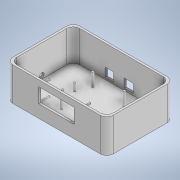
# Autodesk Inventor part: krabička
Saved by Autodesk Inventor 2021 (Build 250183000, 183)
## iProperties
Created: 2020-12-02
Part Number: krabička
Material: Všeobecné
Document SubType Name: Modeling
Designer: Adam
Density: 1 g/cm^3
Appearance: Výchozí
Author: Adam
Autodesk Inventor part; units mm, degrees
ref_plane "YZ Plane" through (0, 0, 0) normal (1, 0, 0) x (0, 1, 0)
ref_plane "XZ Plane" through (0, 0, 0) normal (0, 1, 0) x (-1, 0, 0)
ref_plane "XY Plane" through (0, 0, 0) normal (0, 0, 1) x (1, 0, 0)
sketch "Náčrt1" plane through (0, 0, 0) normal (0, 1, 0) x (-1, 0, 0)
  line L0 (0, 0) -> (-150, 0)
  line L1 (-150, 0) -> (-150, -100)
  line L2 (-150, -100) -> (0, -100)
  line L3 (0, -100) -> (0, 0)
  dimension "d0" = 150
  dimension "d1" = 100
  constraints: 8 end point, 2 parallel, 1 horizontal, 1 perpendicular
  measures "d0" distance of L1.end L2.end
  measures "d1" distance of L0.end L1.end
extrude "Vysunutí1" add sketch "Náčrt1" along normal blind 50
sketch "Náčrt2" plane through (0, 50, 0) normal (0, 1, 0) x (1, 0, 0)
  line L0 (3, 97) -> (147, 97)
  line L1 (147, 97) -> (147, 3)
  line L2 (147, 3) -> (3, 3)
  line L3 (3, 3) -> (3, 97)
  line L4 (0, 100) -> (0, 0) projected
  line L5 (150, 100) -> (0, 100) projected
  dimension "d4" = 144
  dimension "d5" = 94
  dimension "d6" = 3
  dimension "d7" = 3
  constraints: 8 end point, 2 parallel, 1 horizontal, 1 perpendicular
  measures "d4" distance of L0.start L0.end
  measures "d5" distance of L0.end L1.end
  measures "d6" distance between parallel lines of L4 L3
  measures "d7" distance between parallel lines of L5 L0
extrude "Vysunutí2" cut sketch "Náčrt2" against normal blind 47
sketch "Náčrt3" plane through (0, 0, 0) normal (0, 0, 1) x (1, 0, 0)
  line L0 (48.5, 41) -> (101.5, 41)
  line L1 (101.5, 41) -> (101.5, 19)
  line L2 (101.5, 19) -> (48.5, 19)
  line L3 (48.5, 19) -> (48.5, 41)
  line L4 (0, 0) -> (0, 50) projected
  line L5 (0, 0) -> (150, 0) projected
  dimension "d10" = 22
  dimension "d11" = 53
  dimension "d12" = 48.5
  dimension "d13" = 19
  constraints: 8 end point, 2 parallel, 1 horizontal, 1 perpendicular
  measures "d10" distance of L0.end L1.end
  measures "d11" distance of L1.end L2.end
  measures "d12" distance between parallel lines of L4 L3
  measures "d13" distance between parallel lines of L5 L2
extrude "Vysunutí3" cut sketch "Náčrt3" against normal blind 3
sketch "Náčrt4" plane through (147, 50, -3) normal (0, 0, -1) x (-1, 0, 0)
  line L0 (37.5, -7.5) -> (103.5, -7.5)
  line L1 (103.5, -7.5) -> (103.5, -34.5)
  line L2 (103.5, -34.5) -> (37.5, -34.5)
  line L3 (37.5, -34.5) -> (37.5, -7.5)
  line L4 (98.5, -9) -> (98.5, -31) projected
  line L5 (98.5, -31) -> (45.5, -31) projected
  circle A0 centre (101, -10) radius 1.5
  circle A1 centre (40, -10) radius 1.5
  circle A2 centre (40, -32) radius 1.5
  circle A3 centre (101, -32) radius 1.5
  line L6 (45.5, -31) -> (45.5, -9) projected
  line L7 (46.5, -10.5) -> (97.5, -10.5)
  line L8 (97.5, -10.5) -> (97.5, -29.5)
  line L9 (97.5, -29.5) -> (46.5, -29.5)
  line L10 (46.5, -29.5) -> (46.5, -10.5)
  line L11 (45.5, -9) -> (98.5, -9) projected
  point P0 (147, -50)
  point P1 (98.5, -37)
  dimension "d16" = 66
  dimension "d17" = 27
  dimension "d19" = 3.5
  dimension "d21" = 3
  dimension "d22" = 3
  dimension "d23" = 3
  dimension "d24" = 3
  dimension "d56" = 1
  dimension "d57" = 1
  dimension "d58" = 1
  dimension "d59" = 1
  dimension "d60" = 1
  dimension "d61" = 1
  dimension "d62" = 1
  dimension "d63" = 1
  dimension "d129" = 1
  dimension "d130" = 51
  dimension "d131" = 19
  dimension "d132" = 1.5
  dimension "d133" = 6
  dimension "d134" = 9
  constraints: 16 end point, 4 centre point, 3 parallel, 2 horizontal, 2 perpendicular
  measures "d16" distance of L0.start L0.end
  measures "d17" distance of L0.end L1.end
  measures "d19" distance between parallel lines of L5 L2
  measures "d21" diameter of A0
  measures "d22" diameter of A1
  measures "d23" diameter of A2
  measures "d24" diameter of A3
  measures "d56" distance edge to line of A0 L0
  measures "d57" distance edge to line of A0 L1
  measures "d58" distance edge to line of A3 L1
  measures "d59" distance edge to line of A3 L2
  measures "d60" distance edge to line of A1 L0
  measures "d61" distance edge to line of A1 L3
  measures "d62" distance edge to line of A2 L3
  measures "d63" distance edge to line of A2 L2
  measures "d129" distance between parallel lines of L6 L10
  measures "d130" distance of L7.start L7.end
  measures "d131" distance of L7.end L8.end
  measures "d132" distance between parallel lines of L7 L11
  measures "d133" distance between parallel lines of L8 L1
  measures "d134" distance between parallel lines of L3 L10
extrude "Vysunutí4" add sketch "Náčrt4" along normal blind 15 contours A0 | A1 | A2 | A3
fillet "Zaoblení1" radius 10 8 edges at (150, 25, 0) (150, 25, -100) (3, 26.5, -97) (0, 25, -100) (0, 25, 0) (3, 26.5, -3) (147, 26.5, -3) (147, 26.5, -97)
sketch "Náčrt7" plane through (0, 3, 0) normal (0, 1, 0) x (1, 0, 0)
  line L0 (137, 3) -> (13, 3) projected
  line L1 (150, 10) -> (150, 90) projected
  line L2 (13, 97) -> (137, 97) projected
  line L3 (101.7363, 91.2274) -> (101.7363, 27.7499)
  line L4 (101.694, 91.4813) -> (101.7363, 91.2274)
  line L5 (101.5882, 91.7141) -> (101.694, 91.4813)
  line L6 (101.44, 91.9257) -> (101.5882, 91.7141)
  line L7 (101.2285, 92.095) -> (101.44, 91.9257)
  line L8 (100.9957, 92.1796) -> (101.2285, 92.095)
  line L9 (100.7206, 92.2219) -> (100.9957, 92.1796)
  line L10 (49.4308, 92.2219) -> (100.7206, 92.2219)
  line L11 (49.1768, 92.1796) -> (49.4308, 92.2219)
  line L12 (48.9441, 92.095) -> (49.1768, 92.1796)
  line L13 (48.7325, 91.9257) -> (48.9441, 92.095)
  line L14 (48.5632, 91.7141) -> (48.7325, 91.9257)
  line L15 (48.4786, 91.4813) -> (48.5632, 91.7141)
  line L16 (48.4363, 91.2274) -> (48.4786, 91.4813)
  line L17 (48.4363, 27.2968) -> (48.4363, 91.3033)
  line L18 (48.4786, 26.967) -> (48.4363, 27.2209)
  line L19 (48.5632, 26.7342) -> (48.4786, 26.967)
  line L20 (48.7325, 26.5226) -> (48.5632, 26.7342)
  line L21 (48.9441, 26.3533) -> (48.7325, 26.5226)
  line L22 (49.1768, 26.2687) -> (48.9441, 26.3533)
  line L23 (49.4308, 26.2264) -> (49.1768, 26.2687)
  line L24 (50.9754, 26.2264) -> (49.4308, 26.2264)
  line L25 (53.5145, 23.6873) -> (50.9754, 26.2264)
  line L26 (86.2836, 23.6873) -> (53.5504, 23.6873)
  line L27 (88.7869, 26.2264) -> (86.2477, 23.6873)
  line L28 (100.2128, 26.2264) -> (88.7869, 26.2264)
  line L29 (101.7363, 27.7499) -> (100.2128, 26.2264)
  line L30 (97.5901, 76.9312) -> (97.593, 76.8751)
  line L31 (97.593, 76.8751) -> (97.5979, 76.8192)
  line L32 (97.5979, 76.8192) -> (97.6047, 76.7635)
  line L33 (97.6047, 76.7635) -> (97.6135, 76.708)
  line L34 (97.6135, 76.708) -> (97.6242, 76.6529)
  line L35 (97.6242, 76.6529) -> (97.6368, 76.5983)
  line L36 (97.6368, 76.5983) -> (97.6514, 76.544)
  line L37 (97.6514, 76.544) -> (97.6678, 76.4904)
  line L38 (97.6678, 76.4904) -> (97.6861, 76.4373)
  line L39 (97.6861, 76.4373) -> (97.7062, 76.3849)
  line L40 (97.7062, 76.3849) -> (97.7281, 76.3332)
  line L41 (97.7281, 76.3332) -> (97.7518, 76.2823)
  line L42 (97.7518, 76.2823) -> (97.7773, 76.2323)
  line L43 (97.7773, 76.2323) -> (97.8045, 76.1832)
  line L44 (97.8045, 76.1832) -> (97.8334, 76.1351)
  line L45 (97.8334, 76.1351) -> (97.864, 76.0881)
  line L46 (97.864, 76.0881) -> (97.8962, 76.0421)
  line L47 (97.8962, 76.0421) -> (97.93, 75.9972)
  line L48 (97.93, 75.9972) -> (97.9653, 75.9536)
  line L49 (97.9653, 75.9536) -> (98.0021, 75.9113)
  line L50 (98.0021, 75.9113) -> (98.0404, 75.8702)
  line L51 (98.0404, 75.8702) -> (98.0801, 75.8305)
  line L52 (98.0801, 75.8305) -> (98.1211, 75.7922)
  line L53 (98.1211, 75.7922) -> (98.1635, 75.7554)
  line L54 (98.1635, 75.7554) -> (98.2071, 75.7201)
  line L55 (98.2071, 75.7201) -> (98.252, 75.6863)
  line L56 (98.252, 75.6863) -> (98.2979, 75.6541)
  line L57 (98.2979, 75.6541) -> (98.345, 75.6235)
  line L58 (98.345, 75.6235) -> (98.3931, 75.5946)
  line L59 (98.3931, 75.5946) -> (98.4422, 75.5674)
  line L60 (98.4422, 75.5674) -> (98.4922, 75.5419)
  line L61 (98.4922, 75.5419) -> (98.5431, 75.5182)
  line L62 (98.5431, 75.5182) -> (98.5948, 75.4963)
  line L63 (98.5948, 75.4963) -> (98.6472, 75.4762)
  line L64 (98.6472, 75.4762) -> (98.7002, 75.4579)
  line L65 (98.7002, 75.4579) -> (98.7539, 75.4415)
  line L66 (98.7539, 75.4415) -> (98.8081, 75.427)
  line L67 (98.8081, 75.427) -> (98.8628, 75.4143)
  line L68 (98.8628, 75.4143) -> (98.9179, 75.4036)
  line L69 (98.9179, 75.4036) -> (98.9734, 75.3948)
  line L70 (98.9734, 75.3948) -> (99.0291, 75.388)
  line L71 (99.0291, 75.388) -> (99.085, 75.3831)
  line L72 (99.085, 75.3831) -> (99.1411, 75.3802)
  line L73 (99.1411, 75.3802) -> (99.1972, 75.3792)
  line L74 (99.1972, 75.3792) -> (99.2529, 75.3802)
  line L75 (99.2529, 75.3802) -> (99.3085, 75.3831)
  line L76 (99.3085, 75.3831) -> (99.364, 75.3879)
  line L77 (99.364, 75.3879) -> (99.4193, 75.3946)
  line L78 (99.4193, 75.3946) -> (99.4744, 75.4033)
  line L79 (99.4744, 75.4033) -> (99.5291, 75.4138)
  line L80 (99.5291, 75.4138) -> (99.5834, 75.4263)
  line L81 (99.5834, 75.4263) -> (99.6373, 75.4406)
  line L82 (99.6373, 75.4406) -> (99.6906, 75.4568)
  line L83 (99.6906, 75.4568) -> (99.7433, 75.4748)
  line L84 (99.7433, 75.4748) -> (99.7954, 75.4946)
  line L85 (99.7954, 75.4946) -> (99.8467, 75.5162)
  line L86 (99.8467, 75.5162) -> (99.8973, 75.5396)
  line L87 (99.8973, 75.5396) -> (99.947, 75.5647)
  line L88 (99.947, 75.5647) -> (99.9959, 75.5916)
  line L89 (99.9959, 75.5916) -> (100.0437, 75.6201)
  line L90 (100.0437, 75.6201) -> (100.0906, 75.6502)
  line L91 (100.0906, 75.6502) -> (100.1364, 75.682)
  line L92 (100.1364, 75.682) -> (100.181, 75.7153)
  line L93 (100.181, 75.7153) -> (100.2245, 75.7501)
  line L94 (100.2245, 75.7501) -> (100.2667, 75.7865)
  line L95 (100.2667, 75.7865) -> (100.3077, 75.8242)
  line L96 (100.3077, 75.8242) -> (100.3473, 75.8634)
  line L97 (100.3473, 75.8634) -> (100.3856, 75.9039)
  line L98 (100.3856, 75.9039) -> (100.4224, 75.9457)
  line L99 (100.4224, 75.9457) -> (100.4577, 75.9888)
  line L100 (100.4577, 75.9888) -> (100.4916, 76.0331)
  line L101 (100.4916, 76.0331) -> (100.5239, 76.0785)
  line L102 (100.5239, 76.0785) -> (100.5545, 76.125)
  line L103 (100.5545, 76.125) -> (100.5836, 76.1725)
  line L104 (100.5836, 76.1725) -> (100.611, 76.2211)
  line L105 (100.611, 76.2211) -> (100.6367, 76.2705)
  line L106 (100.6367, 76.2705) -> (100.6607, 76.3208)
  line L107 (100.6607, 76.3208) -> (100.6829, 76.3719)
  line L108 (100.6829, 76.3719) -> (100.7033, 76.4237)
  line L109 (100.7033, 76.4237) -> (100.7219, 76.4763)
  line L110 (100.7219, 76.4763) -> (100.7387, 76.5294)
  line L111 (100.7387, 76.5294) -> (100.7536, 76.5831)
  line L112 (100.7536, 76.5831) -> (100.7667, 76.6372)
  line L113 (100.7667, 76.6372) -> (100.7779, 76.6918)
  line L114 (100.7779, 76.6918) -> (100.7872, 76.7467)
  line L115 (100.7872, 76.7467) -> (100.7946, 76.802)
  line L116 (100.7946, 76.802) -> (100.8, 76.8574)
  line L117 (100.8, 76.8574) -> (100.8036, 76.913)
  line L118 (100.8036, 76.913) -> (100.8052, 76.9687)
  line L119 (100.8052, 76.9687) -> (100.8048, 77.0244)
  line L120 (100.8048, 77.0244) -> (100.8026, 77.0801)
  line L121 (100.8026, 77.0801) -> (100.7984, 77.1357)
  line L122 (100.7984, 77.1357) -> (100.7923, 77.1911)
  line L123 (100.7923, 77.1911) -> (100.7843, 77.2462)
  line L124 (100.7843, 77.2462) -> (100.7744, 77.301)
  line L125 (100.7744, 77.301) -> (100.7626, 77.3555)
  line L126 (100.7626, 77.3555) -> (100.7489, 77.4095)
  line L127 (100.7489, 77.4095) -> (100.7333, 77.463)
  line L128 (100.7333, 77.463) -> (100.7159, 77.5159)
  line L129 (100.7159, 77.5159) -> (100.6967, 77.5682)
  line L130 (100.6967, 77.5682) -> (100.6757, 77.6198)
  line L131 (100.6757, 77.6198) -> (100.6529, 77.6706)
  line L132 (100.6529, 77.6706) -> (100.6283, 77.7207)
  line L133 (100.6283, 77.7207) -> (100.602, 77.7698)
  line L134 (100.602, 77.7698) -> (100.5741, 77.818)
  line L135 (100.5741, 77.818) -> (100.5445, 77.8652)
  line L136 (100.5445, 77.8652) -> (100.5133, 77.9113)
  line L137 (100.5133, 77.9113) -> (100.4805, 77.9564)
  line L138 (100.4805, 77.9564) -> (100.4461, 78.0003)
  line L139 (100.4461, 78.0003) -> (100.4103, 78.0429)
  line L140 (100.4103, 78.0429) -> (100.373, 78.0843)
  line L141 (100.373, 78.0843) -> (100.3343, 78.1244)
  line L142 (100.3343, 78.1244) -> (100.2942, 78.1631)
  line L143 (100.2942, 78.1631) -> (100.2528, 78.2004)
  line L144 (100.2528, 78.2004) -> (100.2101, 78.2362)
  line L145 (100.2101, 78.2362) -> (100.1663, 78.2706)
  line L146 (100.1663, 78.2706) -> (100.1212, 78.3034)
  line L147 (100.1212, 78.3034) -> (100.0751, 78.3346)
  line L148 (100.0751, 78.3346) -> (100.0279, 78.3642)
  line L149 (100.0279, 78.3642) -> (99.9797, 78.3922)
  line L150 (99.9797, 78.3922) -> (99.9305, 78.4184)
  line L151 (99.9305, 78.4184) -> (99.8805, 78.443)
  line L152 (99.8805, 78.443) -> (99.8297, 78.4658)
  line L153 (99.8297, 78.4658) -> (99.7781, 78.4868)
  line L154 (99.7781, 78.4868) -> (99.7258, 78.506)
  line L155 (99.7258, 78.506) -> (99.6729, 78.5234)
  line L156 (99.6729, 78.5234) -> (99.6194, 78.539)
  line L157 (99.6194, 78.539) -> (99.5653, 78.5527)
  line L158 (99.5653, 78.5527) -> (99.5109, 78.5645)
  line L159 (99.5109, 78.5645) -> (99.4561, 78.5744)
  line L160 (99.4561, 78.5744) -> (99.4009, 78.5824)
  line L161 (99.4009, 78.5824) -> (99.3455, 78.5885)
  line L162 (99.3455, 78.5885) -> (99.29, 78.5927)
  line L163 (99.29, 78.5927) -> (99.2343, 78.595)
  line L164 (99.2343, 78.595) -> (99.1786, 78.5953)
  line L165 (99.1786, 78.5953) -> (99.1229, 78.5937)
  line L166 (99.1229, 78.5937) -> (99.0673, 78.5901)
  line L167 (99.0673, 78.5901) -> (99.0119, 78.5847)
  line L168 (99.0119, 78.5847) -> (98.9566, 78.5773)
  line L169 (98.9566, 78.5773) -> (98.9017, 78.568)
  line L170 (98.9017, 78.568) -> (98.8471, 78.5568)
  line L171 (98.8471, 78.5568) -> (98.7929, 78.5438)
  line L172 (98.7929, 78.5438) -> (98.7393, 78.5288)
  line L173 (98.7393, 78.5288) -> (98.6861, 78.512)
  line L174 (98.6861, 78.512) -> (98.6336, 78.4934)
  line L175 (98.6336, 78.4934) -> (98.5818, 78.473)
  line L176 (98.5818, 78.473) -> (98.5307, 78.4508)
  line L177 (98.5307, 78.4508) -> (98.4804, 78.4268)
  line L178 (98.4804, 78.4268) -> (98.4309, 78.4011)
  line L179 (98.4309, 78.4011) -> (98.3824, 78.3737)
  line L180 (98.3824, 78.3737) -> (98.3349, 78.3447)
  line L181 (98.3349, 78.3447) -> (98.2884, 78.314)
  line L182 (98.2884, 78.314) -> (98.243, 78.2817)
  line L183 (98.243, 78.2817) -> (98.1987, 78.2479)
  line L184 (98.1987, 78.2479) -> (98.1556, 78.2125)
  line L185 (98.1556, 78.2125) -> (98.1138, 78.1757)
  line L186 (98.1138, 78.1757) -> (98.0733, 78.1374)
  line L187 (98.0733, 78.1374) -> (98.0341, 78.0978)
  line L188 (98.0341, 78.0978) -> (97.9963, 78.0569)
  line L189 (97.9963, 78.0569) -> (97.96, 78.0146)
  line L190 (97.96, 78.0146) -> (97.9252, 77.9711)
  line L191 (97.9252, 77.9711) -> (97.8918, 77.9265)
  line L192 (97.8918, 77.9265) -> (97.8601, 77.8807)
  line L193 (97.8601, 77.8807) -> (97.8299, 77.8338)
  line L194 (97.8299, 77.8338) -> (97.8014, 77.786)
  line L195 (97.8014, 77.786) -> (97.7746, 77.7371)
  line L196 (97.7746, 77.7371) -> (97.7495, 77.6874)
  line L197 (97.7495, 77.6874) -> (97.7261, 77.6368)
  line L198 (97.7261, 77.6368) -> (97.7045, 77.5855)
  line L199 (97.7045, 77.5855) -> (97.6846, 77.5334)
  line L200 (97.6846, 77.5334) -> (97.6666, 77.4807)
  line L201 (97.6666, 77.4807) -> (97.6505, 77.4274)
  line L202 (97.6505, 77.4274) -> (97.6361, 77.3735)
  line L203 (97.6361, 77.3735) -> (97.6237, 77.3192)
  line L204 (97.6237, 77.3192) -> (97.6131, 77.2645)
  line L205 (97.6131, 77.2645) -> (97.6045, 77.2095)
  line L206 (97.6045, 77.2095) -> (97.5978, 77.1542)
  line L207 (97.5978, 77.1542) -> (97.5929, 77.0986)
  line L208 (97.5929, 77.0986) -> (97.59, 77.043)
  line L209 (97.59, 77.043) -> (97.5891, 76.9873)
  line L210 (97.5891, 76.9873) -> (97.5901, 76.9312)
  line L211 (82.3554, 26.1703) -> (82.3584, 26.1142)
  line L212 (82.3584, 26.1142) -> (82.3633, 26.0583)
  line L213 (82.3633, 26.0583) -> (82.3701, 26.0026)
  line L214 (82.3701, 26.0026) -> (82.3789, 25.9472)
  line L215 (82.3789, 25.9472) -> (82.3896, 25.8921)
  line L216 (82.3896, 25.8921) -> (82.4022, 25.8374)
  line L217 (82.4022, 25.8374) -> (82.4168, 25.7831)
  line L218 (82.4168, 25.7831) -> (82.4332, 25.7295)
  line L219 (82.4332, 25.7295) -> (82.4514, 25.6764)
  line L220 (82.4514, 25.6764) -> (82.4716, 25.624)
  line L221 (82.4716, 25.624) -> (82.4935, 25.5723)
  line L222 (82.4935, 25.5723) -> (82.5172, 25.5214)
  line L223 (82.5172, 25.5214) -> (82.5427, 25.4714)
  line L224 (82.5427, 25.4714) -> (82.5699, 25.4223)
  line L225 (82.5699, 25.4223) -> (82.5988, 25.3742)
  line L226 (82.5988, 25.3742) -> (82.6294, 25.3272)
  line L227 (82.6294, 25.3272) -> (82.6616, 25.2812)
  line L228 (82.6616, 25.2812) -> (82.6954, 25.2363)
  line L229 (82.6954, 25.2363) -> (82.7307, 25.1927)
  line L230 (82.7307, 25.1927) -> (82.7675, 25.1504)
  line L231 (82.7675, 25.1504) -> (82.8058, 25.1093)
  line L232 (82.8058, 25.1093) -> (82.8455, 25.0696)
  line L233 (82.8455, 25.0696) -> (82.8865, 25.0313)
  line L234 (82.8865, 25.0313) -> (82.9289, 24.9945)
  line L235 (82.9289, 24.9945) -> (82.9725, 24.9592)
  line L236 (82.9725, 24.9592) -> (83.0173, 24.9254)
  line L237 (83.0173, 24.9254) -> (83.0633, 24.8932)
  line L238 (83.0633, 24.8932) -> (83.1104, 24.8626)
  line L239 (83.1104, 24.8626) -> (83.1585, 24.8337)
  line L240 (83.1585, 24.8337) -> (83.2076, 24.8065)
  line L241 (83.2076, 24.8065) -> (83.2576, 24.781)
  line L242 (83.2576, 24.781) -> (83.3085, 24.7573)
  line L243 (83.3085, 24.7573) -> (83.3602, 24.7354)
  line L244 (83.3602, 24.7354) -> (83.4126, 24.7153)
  line L245 (83.4126, 24.7153) -> (83.4656, 24.697)
  line L246 (83.4656, 24.697) -> (83.5193, 24.6806)
  line L247 (83.5193, 24.6806) -> (83.5735, 24.6661)
  line L248 (83.5735, 24.6661) -> (83.6282, 24.6534)
  line L249 (83.6282, 24.6534) -> (83.6833, 24.6427)
  line L250 (83.6833, 24.6427) -> (83.7388, 24.6339)
  line L251 (83.7388, 24.6339) -> (83.7945, 24.6271)
  line L252 (83.7945, 24.6271) -> (83.8504, 24.6222)
  line L253 (83.8504, 24.6222) -> (83.9064, 24.6193)
  line L254 (83.9064, 24.6193) -> (83.9626, 24.6183)
  line L255 (83.9626, 24.6183) -> (84.0183, 24.6193)
  line L256 (84.0183, 24.6193) -> (84.0739, 24.6222)
  line L257 (84.0739, 24.6222) -> (84.1294, 24.627)
  line L258 (84.1294, 24.627) -> (84.1847, 24.6337)
  line L259 (84.1847, 24.6337) -> (84.2398, 24.6424)
  line L260 (84.2398, 24.6424) -> (84.2945, 24.6529)
  line L261 (84.2945, 24.6529) -> (84.3488, 24.6654)
  line L262 (84.3488, 24.6654) -> (84.4026, 24.6797)
  line L263 (84.4026, 24.6797) -> (84.456, 24.6959)
  line L264 (84.456, 24.6959) -> (84.5087, 24.7139)
  line L265 (84.5087, 24.7139) -> (84.5607, 24.7337)
  line L266 (84.5607, 24.7337) -> (84.6121, 24.7553)
  line L267 (84.6121, 24.7553) -> (84.6627, 24.7787)
  line L268 (84.6627, 24.7787) -> (84.7124, 24.8038)
  line L269 (84.7124, 24.8038) -> (84.7612, 24.8307)
  line L270 (84.7612, 24.8307) -> (84.8091, 24.8592)
  line L271 (84.8091, 24.8592) -> (84.856, 24.8893)
  line L272 (84.856, 24.8893) -> (84.9018, 24.9211)
  line L273 (84.9018, 24.9211) -> (84.9464, 24.9544)
  line L274 (84.9464, 24.9544) -> (84.9899, 24.9892)
  line L275 (84.9899, 24.9892) -> (85.0321, 25.0256)
  line L276 (85.0321, 25.0256) -> (85.0731, 25.0633)
  line L277 (85.0731, 25.0633) -> (85.1127, 25.1025)
  line L278 (85.1127, 25.1025) -> (85.151, 25.143)
  line L279 (85.151, 25.143) -> (85.1878, 25.1848)
  line L280 (85.1878, 25.1848) -> (85.2231, 25.2279)
  line L281 (85.2231, 25.2279) -> (85.257, 25.2722)
  line L282 (85.257, 25.2722) -> (85.2892, 25.3176)
  line L283 (85.2892, 25.3176) -> (85.3199, 25.3641)
  line L284 (85.3199, 25.3641) -> (85.349, 25.4116)
  line L285 (85.349, 25.4116) -> (85.3764, 25.4602)
  line L286 (85.3764, 25.4602) -> (85.4021, 25.5096)
  line L287 (85.4021, 25.5096) -> (85.426, 25.5599)
  line L288 (85.426, 25.5599) -> (85.4482, 25.611)
  line L289 (85.4482, 25.611) -> (85.4687, 25.6628)
  line L290 (85.4687, 25.6628) -> (85.4873, 25.7154)
  line L291 (85.4873, 25.7154) -> (85.5041, 25.7685)
  line L292 (85.5041, 25.7685) -> (85.519, 25.8222)
  line L293 (85.519, 25.8222) -> (85.5321, 25.8763)
  line L294 (85.5321, 25.8763) -> (85.5433, 25.9309)
  line L295 (85.5433, 25.9309) -> (85.5526, 25.9858)
  line L296 (85.5526, 25.9858) -> (85.5599, 26.0411)
  line L297 (85.5599, 26.0411) -> (85.5654, 26.0965)
  line L298 (85.5654, 26.0965) -> (85.5689, 26.1521)
  line L299 (85.5689, 26.1521) -> (85.5705, 26.2078)
  line L300 (85.5705, 26.2078) -> (85.5702, 26.2635)
  line L301 (85.5702, 26.2635) -> (85.568, 26.3192)
  line L302 (85.568, 26.3192) -> (85.5638, 26.3748)
  line L303 (85.5638, 26.3748) -> (85.5577, 26.4302)
  line L304 (85.5577, 26.4302) -> (85.5497, 26.4853)
  line L305 (85.5497, 26.4853) -> (85.5398, 26.5401)
  line L306 (85.5398, 26.5401) -> (85.5279, 26.5946)
  line L307 (85.5279, 26.5946) -> (85.5142, 26.6486)
  line L308 (85.5142, 26.6486) -> (85.4987, 26.7021)
  line L309 (85.4987, 26.7021) -> (85.4813, 26.755)
  line L310 (85.4813, 26.755) -> (85.4621, 26.8073)
  line L311 (85.4621, 26.8073) -> (85.441, 26.8589)
  line L312 (85.441, 26.8589) -> (85.4182, 26.9097)
  line L313 (85.4182, 26.9097) -> (85.3937, 26.9598)
  line L314 (85.3937, 26.9598) -> (85.3674, 27.0089)
  line L315 (85.3674, 27.0089) -> (85.3395, 27.0571)
  line L316 (85.3395, 27.0571) -> (85.3099, 27.1043)
  line L317 (85.3099, 27.1043) -> (85.2786, 27.1505)
  line L318 (85.2786, 27.1505) -> (85.2458, 27.1955)
  line L319 (85.2458, 27.1955) -> (85.2115, 27.2394)
  line L320 (85.2115, 27.2394) -> (85.1757, 27.282)
  line L321 (85.1757, 27.282) -> (85.1384, 27.3234)
  line L322 (85.1384, 27.3234) -> (85.0997, 27.3635)
  line L323 (85.0997, 27.3635) -> (85.0596, 27.4022)
  line L324 (85.0596, 27.4022) -> (85.0182, 27.4395)
  line L325 (85.0182, 27.4395) -> (84.9755, 27.4753)
  line L326 (84.9755, 27.4753) -> (84.9317, 27.5097)
  line L327 (84.9317, 27.5097) -> (84.8866, 27.5425)
  line L328 (84.8866, 27.5425) -> (84.8405, 27.5737)
  line L329 (84.8405, 27.5737) -> (84.7933, 27.6033)
  line L330 (84.7933, 27.6033) -> (84.7451, 27.6313)
  line L331 (84.7451, 27.6313) -> (84.6959, 27.6575)
  line L332 (84.6959, 27.6575) -> (84.6459, 27.6821)
  line L333 (82.3545, 26.2264) -> (82.3554, 26.1703)
  line L334 (84.5951, 27.7049) -> (84.5435, 27.7259)
  line L335 (84.5435, 27.7259) -> (84.4912, 27.7451)
  line L336 (84.4912, 27.7451) -> (84.4382, 27.7625)
  line L337 (84.4382, 27.7625) -> (84.3847, 27.7781)
  line L338 (84.3847, 27.7781) -> (84.3307, 27.7918)
  line L339 (84.3307, 27.7918) -> (84.2763, 27.8036)
  line L340 (84.2763, 27.8036) -> (84.2215, 27.8135)
  line L341 (84.2215, 27.8135) -> (84.1663, 27.8215)
  line L342 (84.1663, 27.8215) -> (84.1109, 27.8276)
  line L343 (84.1109, 27.8276) -> (84.0554, 27.8318)
  line L344 (84.0554, 27.8318) -> (83.9997, 27.8341)
  line L345 (83.9997, 27.8341) -> (83.944, 27.8344)
  line L346 (83.944, 27.8344) -> (83.8883, 27.8328)
  line L347 (83.8883, 27.8328) -> (83.8327, 27.8292)
  line L348 (83.8327, 27.8292) -> (83.7772, 27.8238)
  line L349 (83.7772, 27.8238) -> (83.722, 27.8164)
  line L350 (83.722, 27.8164) -> (83.6671, 27.8071)
  line L351 (83.6671, 27.8071) -> (83.6125, 27.7959)
  line L352 (83.6125, 27.7959) -> (83.5583, 27.7829)
  line L353 (83.5583, 27.7829) -> (83.5046, 27.7679)
  line L354 (83.5046, 27.7679) -> (83.4515, 27.7511)
  line L355 (83.4515, 27.7511) -> (83.399, 27.7325)
  line L356 (83.399, 27.7325) -> (83.3472, 27.7121)
  line L357 (83.3472, 27.7121) -> (83.2961, 27.6899)
  line L358 (83.2961, 27.6899) -> (83.2458, 27.6659)
  line L359 (83.2458, 27.6659) -> (83.1963, 27.6402)
  line L360 (83.1963, 27.6402) -> (83.1478, 27.6128)
  line L361 (83.1478, 27.6128) -> (83.1003, 27.5838)
  line L362 (83.1003, 27.5838) -> (83.0538, 27.5531)
  line L363 (83.0538, 27.5531) -> (83.0083, 27.5208)
  line L364 (83.0083, 27.5208) -> (82.9641, 27.487)
  line L365 (82.9641, 27.487) -> (82.921, 27.4516)
  line L366 (82.921, 27.4516) -> (82.8792, 27.4148)
  line L367 (82.8792, 27.4148) -> (82.8387, 27.3765)
  line L368 (82.8387, 27.3765) -> (82.7995, 27.3369)
  line L369 (82.7995, 27.3369) -> (82.7617, 27.296)
  line L370 (82.7617, 27.296) -> (82.7254, 27.2537)
  line L371 (82.7254, 27.2537) -> (82.6905, 27.2102)
  line L372 (82.6905, 27.2102) -> (82.6572, 27.1656)
  line L373 (82.6572, 27.1656) -> (82.6255, 27.1198)
  line L374 (82.6255, 27.1198) -> (82.5953, 27.0729)
  line L375 (82.5953, 27.0729) -> (82.5668, 27.0251)
  line L376 (82.5668, 27.0251) -> (82.54, 26.9762)
  line L377 (82.54, 26.9762) -> (82.5149, 26.9265)
  line L378 (82.5149, 26.9265) -> (82.4915, 26.8759)
  line L379 (82.4915, 26.8759) -> (82.4699, 26.8246)
  line L380 (82.4699, 26.8246) -> (82.45, 26.7725)
  line L381 (82.45, 26.7725) -> (82.432, 26.7198)
  line L382 (82.432, 26.7198) -> (82.4158, 26.6665)
  line L383 (82.4158, 26.6665) -> (82.4015, 26.6126)
  line L384 (82.4015, 26.6126) -> (82.3891, 26.5583)
  line L385 (82.3891, 26.5583) -> (82.3785, 26.5036)
  line L386 (82.3785, 26.5036) -> (82.3699, 26.4486)
  line L387 (82.3699, 26.4486) -> (82.3631, 26.3933)
  line L388 (82.3631, 26.3933) -> (82.3583, 26.3377)
  line L389 (82.3583, 26.3377) -> (82.3554, 26.2821)
  line L390 (82.3554, 26.2821) -> (82.3545, 26.2264)
  line L391 (49.3673, 78.2568) -> (49.3683, 78.2007)
  line L392 (49.3683, 78.2007) -> (49.3712, 78.1447)
  line L393 (49.3712, 78.1447) -> (49.3761, 78.0888)
  line L394 (49.3761, 78.0888) -> (49.3829, 78.033)
  line L395 (49.3829, 78.033) -> (49.3917, 77.9776)
  line L396 (49.3917, 77.9776) -> (49.4024, 77.9225)
  line L397 (49.4024, 77.9225) -> (49.415, 77.8678)
  line L398 (49.415, 77.8678) -> (49.4296, 77.8136)
  line L399 (49.4296, 77.8136) -> (49.446, 77.7599)
  line L400 (49.446, 77.7599) -> (49.4643, 77.7068)
  line L401 (49.4643, 77.7068) -> (49.4844, 77.6544)
  line L402 (49.4844, 77.6544) -> (49.5063, 77.6028)
  line L403 (49.5063, 77.6028) -> (49.53, 77.5519)
  line L404 (49.53, 77.5519) -> (49.5555, 77.5019)
  line L405 (49.5555, 77.5019) -> (49.5827, 77.4528)
  line L406 (49.5827, 77.4528) -> (49.6116, 77.4047)
  line L407 (49.6116, 77.4047) -> (49.6422, 77.3576)
  line L408 (49.6422, 77.3576) -> (49.6744, 77.3116)
  line L409 (49.6744, 77.3116) -> (49.7082, 77.2668)
  line L410 (49.7082, 77.2668) -> (49.7435, 77.2232)
  line L411 (49.7435, 77.2232) -> (49.7803, 77.1808)
  line L412 (49.7803, 77.1808) -> (49.8186, 77.1398)
  line L413 (49.8186, 77.1398) -> (49.8583, 77.1001)
  line L414 (49.8583, 77.1001) -> (49.8994, 77.0618)
  line L415 (49.8994, 77.0618) -> (49.9417, 77.025)
  line L416 (49.9417, 77.025) -> (49.9853, 76.9896)
  line L417 (49.9853, 76.9896) -> (50.0302, 76.9559)
  line L418 (50.0302, 76.9559) -> (50.0761, 76.9237)
  line L419 (50.0761, 76.9237) -> (50.1232, 76.8931)
  line L420 (50.1232, 76.8931) -> (50.1713, 76.8642)
  line L421 (50.1713, 76.8642) -> (50.2204, 76.837)
  line L422 (50.2204, 76.837) -> (50.2704, 76.8115)
  line L423 (50.2704, 76.8115) -> (50.3213, 76.7878)
  line L424 (50.3213, 76.7878) -> (50.373, 76.7658)
  line L425 (50.373, 76.7658) -> (50.4254, 76.7457)
  line L426 (50.4254, 76.7457) -> (50.4784, 76.7274)
  line L427 (50.4784, 76.7274) -> (50.5321, 76.711)
  line L428 (50.5321, 76.711) -> (50.5863, 76.6965)
  line L429 (50.5863, 76.6965) -> (50.641, 76.6839)
  line L430 (50.641, 76.6839) -> (50.6961, 76.6732)
  line L431 (50.6961, 76.6732) -> (50.7516, 76.6644)
  line L432 (50.7516, 76.6644) -> (50.8073, 76.6576)
  line L433 (50.8073, 76.6576) -> (50.8632, 76.6527)
  line L434 (50.8632, 76.6527) -> (50.9193, 76.6497)
  line L435 (50.9193, 76.6497) -> (50.9754, 76.6487)
  line L436 (50.9754, 76.6487) -> (51.0311, 76.6497)
  line L437 (51.0311, 76.6497) -> (51.0867, 76.6526)
  line L438 (51.0867, 76.6526) -> (51.1422, 76.6574)
  line L439 (51.1422, 76.6574) -> (51.1975, 76.6642)
  line L440 (51.1975, 76.6642) -> (51.2526, 76.6728)
  line L441 (51.2526, 76.6728) -> (51.3073, 76.6834)
  line L442 (51.3073, 76.6834) -> (51.3616, 76.6958)
  line L443 (51.3616, 76.6958) -> (51.4155, 76.7101)
  line L444 (51.4155, 76.7101) -> (51.4688, 76.7263)
  line L445 (51.4688, 76.7263) -> (51.5215, 76.7443)
  line L446 (51.5215, 76.7443) -> (51.5736, 76.7641)
  line L447 (51.5736, 76.7641) -> (51.6249, 76.7858)
  line L448 (51.6249, 76.7858) -> (51.6755, 76.8091)
  line L449 (51.6755, 76.8091) -> (51.7252, 76.8343)
  line L450 (51.7252, 76.8343) -> (51.7741, 76.8611)
  line L451 (51.7741, 76.8611) -> (51.8219, 76.8896)
  line L452 (51.8219, 76.8896) -> (51.8688, 76.9198)
  line L453 (51.8688, 76.9198) -> (51.9146, 76.9515)
  line L454 (51.9146, 76.9515) -> (51.9592, 76.9848)
  line L455 (51.9592, 76.9848) -> (52.0027, 77.0197)
  line L456 (52.0027, 77.0197) -> (52.0449, 77.056)
  line L457 (52.0449, 77.056) -> (52.0859, 77.0938)
  line L458 (52.0859, 77.0938) -> (52.1255, 77.133)
  line L459 (52.1255, 77.133) -> (52.1638, 77.1735)
  line L460 (52.1638, 77.1735) -> (52.2006, 77.2153)
  line L461 (52.2006, 77.2153) -> (52.2359, 77.2584)
  line L462 (52.2359, 77.2584) -> (52.2698, 77.3026)
  line L463 (52.2698, 77.3026) -> (52.3021, 77.348)
  line L464 (52.3021, 77.348) -> (52.3327, 77.3946)
  line L465 (52.3327, 77.3946) -> (52.3618, 77.4421)
  line L466 (52.3618, 77.4421) -> (52.3892, 77.4906)
  line L467 (52.3892, 77.4906) -> (52.4149, 77.5401)
  line L468 (52.4149, 77.5401) -> (52.4389, 77.5904)
  line L469 (52.4389, 77.5904) -> (52.4611, 77.6414)
  line L470 (52.4611, 77.6414) -> (52.4815, 77.6933)
  line L471 (52.4815, 77.6933) -> (52.5001, 77.7458)
  line L472 (52.5001, 77.7458) -> (52.5169, 77.7989)
  line L473 (52.5169, 77.7989) -> (52.5318, 77.8526)
  line L474 (52.5318, 77.8526) -> (52.5449, 77.9068)
  line L475 (52.5449, 77.9068) -> (52.5561, 77.9614)
  line L476 (52.5561, 77.9614) -> (52.5654, 78.0163)
  line L477 (52.5654, 78.0163) -> (52.5728, 78.0715)
  line L478 (52.5728, 78.0715) -> (52.5782, 78.127)
  line L479 (52.5782, 78.127) -> (52.5818, 78.1826)
  line L480 (52.5818, 78.1826) -> (52.5834, 78.2383)
  line L481 (52.5834, 78.2383) -> (52.583, 78.294)
  line L482 (52.583, 78.294) -> (52.5808, 78.3497)
  line L483 (52.5808, 78.3497) -> (52.5766, 78.4052)
  line L484 (52.5766, 78.4052) -> (52.5705, 78.4606)
  line L485 (52.5705, 78.4606) -> (52.5625, 78.5157)
  line L486 (52.5625, 78.5157) -> (52.5526, 78.5706)
  line L487 (52.5526, 78.5706) -> (52.5408, 78.625)
  line L488 (52.5408, 78.625) -> (52.5271, 78.679)
  line L489 (52.5271, 78.679) -> (52.5115, 78.7325)
  line L490 (52.5115, 78.7325) -> (52.4941, 78.7855)
  line L491 (52.4941, 78.7855) -> (52.4749, 78.8378)
  line L492 (52.4749, 78.8378) -> (52.4539, 78.8894)
  line L493 (52.4539, 78.8894) -> (52.4311, 78.9402)
  line L494 (52.4311, 78.9402) -> (52.4065, 78.9902)
  line L495 (52.4065, 78.9902) -> (52.3802, 79.0394)
  line L496 (52.3802, 79.0394) -> (52.3523, 79.0875)
  line L497 (52.3523, 79.0875) -> (52.3227, 79.1348)
  line L498 (52.3227, 79.1348) -> (52.2915, 79.1809)
  line L499 (52.2915, 79.1809) -> (52.2587, 79.2259)
  line L500 (52.2587, 79.2259) -> (52.2243, 79.2698)
  line L501 (52.2243, 79.2698) -> (52.1885, 79.3125)
  line L502 (52.1885, 79.3125) -> (52.1512, 79.3539)
  line L503 (52.1512, 79.3539) -> (52.1125, 79.3939)
  line L504 (52.1125, 79.3939) -> (52.0724, 79.4326)
  line L505 (52.0724, 79.4326) -> (52.031, 79.4699)
  line L506 (52.031, 79.4699) -> (51.9884, 79.5058)
  line L507 (51.9884, 79.5058) -> (51.9445, 79.5401)
  line L508 (51.9445, 79.5401) -> (51.8994, 79.5729)
  line L509 (51.8994, 79.5729) -> (51.8533, 79.6042)
  line L510 (51.8533, 79.6042) -> (51.8061, 79.6338)
  line L511 (51.8061, 79.6338) -> (51.7579, 79.6617)
  line L512 (51.7579, 79.6617) -> (51.7087, 79.688)
  line L513 (51.7087, 79.688) -> (51.6587, 79.7125)
  line L514 (51.6587, 79.7125) -> (51.6079, 79.7353)
  line L515 (51.6079, 79.7353) -> (51.5563, 79.7563)
  line L516 (51.5563, 79.7563) -> (51.504, 79.7756)
  line L517 (51.504, 79.7756) -> (51.4511, 79.793)
  line L518 (51.4511, 79.793) -> (51.3976, 79.8085)
  line L519 (51.3976, 79.8085) -> (51.3436, 79.8222)
  line L520 (51.3436, 79.8222) -> (51.2891, 79.834)
  line L521 (51.2891, 79.834) -> (51.2343, 79.844)
  line L522 (51.2343, 79.844) -> (51.1791, 79.852)
  line L523 (51.1791, 79.852) -> (51.1238, 79.8581)
  line L524 (51.1238, 79.8581) -> (51.0682, 79.8623)
  line L525 (51.0682, 79.8623) -> (51.0125, 79.8645)
  line L526 (51.0125, 79.8645) -> (50.9568, 79.8648)
  line L527 (50.9568, 79.8648) -> (50.9011, 79.8632)
  line L528 (50.9011, 79.8632) -> (50.8455, 79.8597)
  line L529 (50.8455, 79.8597) -> (50.7901, 79.8542)
  line L530 (50.7901, 79.8542) -> (50.7348, 79.8468)
  line L531 (50.7348, 79.8468) -> (50.6799, 79.8376)
  line L532 (50.6799, 79.8376) -> (50.6253, 79.8264)
  line L533 (50.6253, 79.8264) -> (50.5711, 79.8133)
  line L534 (50.5711, 79.8133) -> (50.5175, 79.7984)
  line L535 (50.5175, 79.7984) -> (50.4643, 79.7816)
  line L536 (50.4643, 79.7816) -> (50.4118, 79.763)
  line L537 (50.4118, 79.763) -> (50.36, 79.7425)
  line L538 (50.36, 79.7425) -> (50.3089, 79.7203)
  line L539 (50.3089, 79.7203) -> (50.2586, 79.6964)
  line L540 (50.2586, 79.6964) -> (50.2091, 79.6707)
  line L541 (50.2091, 79.6707) -> (50.1606, 79.6433)
  line L542 (50.1606, 79.6433) -> (50.1131, 79.6142)
  line L543 (84.6459, 27.6821) -> (84.5951, 27.7049)
  line L544 (50.0666, 79.5835) -> (50.0212, 79.5512)
  line L545 (50.0212, 79.5512) -> (49.9769, 79.5174)
  line L546 (49.9769, 79.5174) -> (49.9338, 79.4821)
  line L547 (49.9338, 79.4821) -> (49.892, 79.4452)
  line L548 (49.892, 79.4452) -> (49.8515, 79.407)
  line L549 (49.8515, 79.407) -> (49.8123, 79.3674)
  line L550 (49.8123, 79.3674) -> (49.7745, 79.3264)
  line L551 (49.7745, 79.3264) -> (49.7382, 79.2842)
  line L552 (49.7382, 79.2842) -> (49.7034, 79.2407)
  line L553 (49.7034, 79.2407) -> (49.67, 79.196)
  line L554 (49.67, 79.196) -> (49.6383, 79.1503)
  line L555 (49.6383, 79.1503) -> (49.6081, 79.1034)
  line L556 (49.6081, 79.1034) -> (49.5796, 79.0555)
  line L557 (49.5796, 79.0555) -> (49.5528, 79.0067)
  line L558 (49.5528, 79.0067) -> (49.5277, 78.957)
  line L559 (49.5277, 78.957) -> (49.5043, 78.9064)
  line L560 (49.5043, 78.9064) -> (49.4827, 78.855)
  line L561 (49.4827, 78.855) -> (49.4629, 78.803)
  line L562 (49.4629, 78.803) -> (49.4448, 78.7502)
  line L563 (49.4448, 78.7502) -> (49.4287, 78.6969)
  line L564 (49.4287, 78.6969) -> (49.4144, 78.6431)
  line L565 (49.4144, 78.6431) -> (49.4019, 78.5888)
  line L566 (49.4019, 78.5888) -> (49.3914, 78.5341)
  line L567 (49.3914, 78.5341) -> (49.3827, 78.479)
  line L568 (49.3827, 78.479) -> (49.376, 78.4237)
  line L569 (49.376, 78.4237) -> (49.3711, 78.3682)
  line L570 (49.3711, 78.3682) -> (49.3682, 78.3126)
  line L571 (49.3682, 78.3126) -> (49.3673, 78.2568)
  line L572 (54.4455, 26.2264) -> (54.4465, 26.1703)
  line L573 (54.4465, 26.1703) -> (54.4494, 26.1142)
  line L574 (54.4494, 26.1142) -> (54.4543, 26.0583)
  line L575 (54.4543, 26.0583) -> (54.4611, 26.0026)
  line L576 (54.4611, 26.0026) -> (54.4699, 25.9472)
  line L577 (54.4699, 25.9472) -> (54.4806, 25.8921)
  line L578 (54.4806, 25.8921) -> (54.4933, 25.8374)
  line L579 (54.4933, 25.8374) -> (54.5078, 25.7831)
  line L580 (54.5078, 25.7831) -> (54.5242, 25.7295)
  line L581 (54.5242, 25.7295) -> (54.5425, 25.6764)
  line L582 (54.5425, 25.6764) -> (54.5626, 25.624)
  line L583 (54.5626, 25.624) -> (54.5845, 25.5723)
  line L584 (54.5845, 25.5723) -> (54.6082, 25.5214)
  line L585 (54.6082, 25.5214) -> (54.6337, 25.4714)
  line L586 (54.6337, 25.4714) -> (54.6609, 25.4223)
  line L587 (54.6609, 25.4223) -> (54.6898, 25.3742)
  line L588 (54.6898, 25.3742) -> (54.7204, 25.3272)
  line L589 (54.7204, 25.3272) -> (54.7526, 25.2812)
  line L590 (54.7526, 25.2812) -> (54.7864, 25.2363)
  line L591 (54.7864, 25.2363) -> (54.8217, 25.1927)
  line L592 (54.8217, 25.1927) -> (54.8585, 25.1504)
  line L593 (54.8585, 25.1504) -> (54.8968, 25.1093)
  line L594 (54.8968, 25.1093) -> (54.9365, 25.0696)
  line L595 (54.9365, 25.0696) -> (54.9776, 25.0313)
  line L596 (54.9776, 25.0313) -> (55.0199, 24.9945)
  line L597 (55.0199, 24.9945) -> (55.0635, 24.9592)
  line L598 (55.0635, 24.9592) -> (55.1084, 24.9254)
  line L599 (55.1084, 24.9254) -> (55.1543, 24.8932)
  line L600 (55.1543, 24.8932) -> (55.2014, 24.8626)
  line L601 (55.2014, 24.8626) -> (55.2495, 24.8337)
  line L602 (55.2495, 24.8337) -> (55.2986, 24.8065)
  line L603 (55.2986, 24.8065) -> (55.3486, 24.781)
  line L604 (55.3486, 24.781) -> (55.3995, 24.7573)
  line L605 (55.3995, 24.7573) -> (55.4512, 24.7354)
  line L606 (55.4512, 24.7354) -> (55.5036, 24.7153)
  line L607 (55.5036, 24.7153) -> (55.5567, 24.697)
  line L608 (55.5567, 24.697) -> (55.6103, 24.6806)
  line L609 (55.6103, 24.6806) -> (55.6646, 24.6661)
  line L610 (55.6646, 24.6661) -> (55.7192, 24.6534)
  line L611 (55.7192, 24.6534) -> (55.7743, 24.6427)
  line L612 (55.7743, 24.6427) -> (55.8298, 24.6339)
  line L613 (55.8298, 24.6339) -> (55.8855, 24.6271)
  line L614 (55.8855, 24.6271) -> (55.9414, 24.6222)
  line L615 (55.9414, 24.6222) -> (55.9975, 24.6193)
  line L616 (55.9975, 24.6193) -> (56.0536, 24.6183)
  line L617 (56.0536, 24.6183) -> (56.1093, 24.6193)
  line L618 (56.1093, 24.6193) -> (56.1649, 24.6222)
  line L619 (56.1649, 24.6222) -> (56.2204, 24.627)
  line L620 (56.2204, 24.627) -> (56.2758, 24.6337)
  line L621 (56.2758, 24.6337) -> (56.3308, 24.6424)
  line L622 (56.3308, 24.6424) -> (56.3855, 24.6529)
  line L623 (56.3855, 24.6529) -> (56.4398, 24.6654)
  line L624 (56.4398, 24.6654) -> (56.4937, 24.6797)
  line L625 (56.4937, 24.6797) -> (56.547, 24.6959)
  line L626 (56.547, 24.6959) -> (56.5997, 24.7139)
  line L627 (56.5997, 24.7139) -> (56.6518, 24.7337)
  line L628 (56.6518, 24.7337) -> (56.7031, 24.7553)
  line L629 (56.7031, 24.7553) -> (56.7537, 24.7787)
  line L630 (56.7537, 24.7787) -> (56.8034, 24.8038)
  line L631 (56.8034, 24.8038) -> (56.8523, 24.8307)
  line L632 (56.8523, 24.8307) -> (56.9001, 24.8592)
  line L633 (56.9001, 24.8592) -> (56.947, 24.8893)
  line L634 (56.947, 24.8893) -> (56.9928, 24.9211)
  line L635 (56.9928, 24.9211) -> (57.0374, 24.9544)
  line L636 (57.0374, 24.9544) -> (57.0809, 24.9892)
  line L637 (57.0809, 24.9892) -> (57.1232, 25.0256)
  line L638 (57.1232, 25.0256) -> (57.1641, 25.0633)
  line L639 (57.1641, 25.0633) -> (57.2037, 25.1025)
  line L640 (57.2037, 25.1025) -> (57.242, 25.143)
  line L641 (57.242, 25.143) -> (57.2788, 25.1848)
  line L642 (57.2788, 25.1848) -> (57.3141, 25.2279)
  line L643 (57.3141, 25.2279) -> (57.348, 25.2722)
  line L644 (57.348, 25.2722) -> (57.3803, 25.3176)
  line L645 (57.3803, 25.3176) -> (57.4109, 25.3641)
  line L646 (57.4109, 25.3641) -> (57.44, 25.4116)
  line L647 (57.44, 25.4116) -> (57.4674, 25.4602)
  line L648 (57.4674, 25.4602) -> (57.4931, 25.5096)
  line L649 (57.4931, 25.5096) -> (57.5171, 25.5599)
  line L650 (57.5171, 25.5599) -> (57.5393, 25.611)
  line L651 (57.5393, 25.611) -> (57.5597, 25.6628)
  line L652 (57.5597, 25.6628) -> (57.5783, 25.7154)
  line L653 (57.5783, 25.7154) -> (57.5951, 25.7685)
  line L654 (57.5951, 25.7685) -> (57.61, 25.8222)
  line L655 (57.61, 25.8222) -> (57.6231, 25.8763)
  line L656 (57.6231, 25.8763) -> (57.6343, 25.9309)
  line L657 (57.6343, 25.9309) -> (57.6436, 25.9858)
  line L658 (57.6436, 25.9858) -> (57.651, 26.0411)
  line L659 (57.651, 26.0411) -> (57.6564, 26.0965)
  line L660 (57.6564, 26.0965) -> (57.66, 26.1521)
  line L661 (57.66, 26.1521) -> (57.6616, 26.2078)
  line L662 (57.6616, 26.2078) -> (57.6613, 26.2635)
  line L663 (57.6613, 26.2635) -> (57.659, 26.3192)
  line L664 (57.659, 26.3192) -> (57.6548, 26.3748)
  line L665 (57.6548, 26.3748) -> (57.6487, 26.4302)
  line L666 (57.6487, 26.4302) -> (57.6407, 26.4853)
  line L667 (57.6407, 26.4853) -> (57.6308, 26.5401)
  line L668 (57.6308, 26.5401) -> (57.619, 26.5946)
  line L669 (57.619, 26.5946) -> (57.6053, 26.6486)
  line L670 (57.6053, 26.6486) -> (57.5897, 26.7021)
  line L671 (57.5897, 26.7021) -> (57.5723, 26.755)
  line L672 (57.5723, 26.755) -> (57.5531, 26.8073)
  line L673 (57.5531, 26.8073) -> (57.5321, 26.8589)
  line L674 (57.5321, 26.8589) -> (57.5093, 26.9097)
  line L675 (57.5093, 26.9097) -> (57.4847, 26.9598)
  line L676 (57.4847, 26.9598) -> (57.4585, 27.0089)
  line L677 (57.4585, 27.0089) -> (57.4305, 27.0571)
  line L678 (57.4305, 27.0571) -> (57.4009, 27.1043)
  line L679 (57.4009, 27.1043) -> (57.3697, 27.1505)
  line L680 (57.3697, 27.1505) -> (57.3369, 27.1955)
  line L681 (57.3369, 27.1955) -> (57.3025, 27.2394)
  line L682 (57.3025, 27.2394) -> (57.2667, 27.282)
  line L683 (57.2667, 27.282) -> (57.2294, 27.3234)
  line L684 (57.2294, 27.3234) -> (57.1907, 27.3635)
  line L685 (57.1907, 27.3635) -> (57.1506, 27.4022)
  line L686 (57.1506, 27.4022) -> (57.1092, 27.4395)
  line L687 (57.1092, 27.4395) -> (57.0666, 27.4753)
  line L688 (57.0666, 27.4753) -> (57.0227, 27.5097)
  line L689 (57.0227, 27.5097) -> (56.9776, 27.5425)
  line L690 (56.9776, 27.5425) -> (56.9315, 27.5737)
  line L691 (56.9315, 27.5737) -> (56.8843, 27.6033)
  line L692 (56.8843, 27.6033) -> (56.8361, 27.6313)
  line L693 (56.8361, 27.6313) -> (56.787, 27.6575)
  line L694 (56.787, 27.6575) -> (56.7369, 27.6821)
  line L695 (56.7369, 27.6821) -> (56.6861, 27.7049)
  line L696 (56.6861, 27.7049) -> (56.6345, 27.7259)
  line L697 (56.6345, 27.7259) -> (56.5822, 27.7451)
  line L698 (56.5822, 27.7451) -> (56.5293, 27.7625)
  line L699 (56.5293, 27.7625) -> (56.4758, 27.7781)
  line L700 (56.4758, 27.7781) -> (56.4218, 27.7918)
  line L701 (56.4218, 27.7918) -> (56.3673, 27.8036)
  line L702 (56.3673, 27.8036) -> (56.3125, 27.8135)
  line L703 (56.3125, 27.8135) -> (56.2573, 27.8215)
  line L704 (56.2573, 27.8215) -> (56.202, 27.8276)
  line L705 (56.202, 27.8276) -> (56.1464, 27.8318)
  line L706 (56.1464, 27.8318) -> (56.0907, 27.8341)
  line L707 (56.0907, 27.8341) -> (56.035, 27.8344)
  line L708 (56.035, 27.8344) -> (55.9793, 27.8328)
  line L709 (55.9793, 27.8328) -> (55.9237, 27.8292)
  line L710 (55.9237, 27.8292) -> (55.8683, 27.8238)
  line L711 (55.8683, 27.8238) -> (55.813, 27.8164)
  line L712 (55.813, 27.8164) -> (55.7581, 27.8071)
  line L713 (55.7581, 27.8071) -> (55.7035, 27.7959)
  line L714 (55.7035, 27.7959) -> (55.6494, 27.7829)
  line L715 (55.6494, 27.7829) -> (55.5957, 27.7679)
  line L716 (55.5957, 27.7679) -> (55.5425, 27.7511)
  line L717 (55.5425, 27.7511) -> (55.49, 27.7325)
  line L718 (55.49, 27.7325) -> (55.4382, 27.7121)
  line L719 (55.4382, 27.7121) -> (55.3871, 27.6899)
  line L720 (55.3871, 27.6899) -> (55.3368, 27.6659)
  line L721 (55.3368, 27.6659) -> (55.2874, 27.6402)
  line L722 (55.2874, 27.6402) -> (55.2388, 27.6128)
  line L723 (55.2388, 27.6128) -> (55.1913, 27.5838)
  line L724 (55.1913, 27.5838) -> (55.1448, 27.5531)
  line L725 (55.1448, 27.5531) -> (55.0994, 27.5208)
  line L726 (55.0994, 27.5208) -> (55.0551, 27.487)
  line L727 (55.0551, 27.487) -> (55.012, 27.4516)
  line L728 (55.012, 27.4516) -> (54.9702, 27.4148)
  line L729 (54.9702, 27.4148) -> (54.9297, 27.3765)
  line L730 (54.9297, 27.3765) -> (54.8905, 27.3369)
  line L731 (54.8905, 27.3369) -> (54.8528, 27.296)
  line L732 (54.8528, 27.296) -> (54.8164, 27.2537)
  line L733 (54.8164, 27.2537) -> (54.7816, 27.2102)
  line L734 (54.7816, 27.2102) -> (54.7483, 27.1656)
  line L735 (54.7483, 27.1656) -> (54.7165, 27.1198)
  line L736 (54.7165, 27.1198) -> (54.6864, 27.0729)
  line L737 (54.6864, 27.0729) -> (54.6578, 27.0251)
  line L738 (54.6578, 27.0251) -> (54.631, 26.9762)
  line L739 (54.631, 26.9762) -> (54.6059, 26.9265)
  line L740 (54.6059, 26.9265) -> (54.5825, 26.8759)
  line L741 (54.5825, 26.8759) -> (54.5609, 26.8246)
  line L742 (54.5609, 26.8246) -> (54.5411, 26.7725)
  line L743 (54.5411, 26.7725) -> (54.523, 26.7198)
  line L744 (54.523, 26.7198) -> (54.5069, 26.6665)
  line L745 (54.5069, 26.6665) -> (54.4926, 26.6126)
  line L746 (54.4926, 26.6126) -> (54.4801, 26.5583)
  line L747 (54.4801, 26.5583) -> (54.4696, 26.5036)
  line L748 (54.4696, 26.5036) -> (54.4609, 26.4486)
  line L749 (54.4609, 26.4486) -> (54.4542, 26.3933)
  line L750 (54.4542, 26.3933) -> (54.4493, 26.3377)
  line L751 (54.4493, 26.3377) -> (54.4465, 26.2821)
  line L752 (54.4465, 26.2821) -> (54.4455, 26.2264)
  line L753 (50.1131, 79.6142) -> (50.0666, 79.5835)
  circle A0 centre (50.954, 78.27) radius 1.5
  circle A1 centre (99.1863, 77) radius 1.5
  circle A2 centre (56.0354, 26.2373) radius 1.5
  circle A3 centre (83.9598, 26.2373) radius 1.5
  point P0 (0, 0)
  dimension "d48" = 3
  dimension "d52" = 3
  dimension "d66" = 1.05
  dimension "d67" = 1.0177
  dimension "d68" = 3
  dimension "d69" = 1.05
  dimension "d70" = 5.06
  dimension "d71" = 3
  dimension "d72" = 1.05
  constraints: 1502 end point, 4 centre point
  measures "d48" diameter of A0
  measures "d52" diameter of A1
  measures "d66" distance edge to line of A1 L3
  measures "d67" distance edge to line of A0 L17
  measures "d68" diameter of A2
  measures "d69" distance edge to line of A2 L26
  measures "d70" distance of A2.centre L24.start
  measures "d71" diameter of A3
  measures "d72" distance edge to line of A3 L26
extrude "Vysunutí6" add sketch "Náčrt7" along normal blind 20 contours A0 | A1 | A2 | A3
sketch "Náčrt10" plane through (13, 50, -97) normal (0, 0, 1) x (1, 0, 0)
  line L0 (0, -47) -> (124, -47) projected
  line L1 (80, -44) -> (66, -44)
  line L2 (66, -44) -> (66, -31)
  line L3 (66, -31) -> (80, -31)
  line L4 (80, -31) -> (80, -44)
  line L5 (124, 0) -> (124, -47) projected
  line L6 (38, -31) -> (50, -31)
  line L7 (50, -31) -> (50, -44)
  line L8 (50, -44) -> (38, -44)
  line L9 (38, -44) -> (38, -31)
  point P0 (-13, -50)
  point P1 (124, -50)
  dimension "d87" = 14
  dimension "d88" = 13
  dimension "d91" = 44
  dimension "d92" = 3
  dimension "d93" = 16
  dimension "d94" = 12
  dimension "d95" = 13
  dimension "d96" = 3
  constraints: 16 end point, 4 parallel, 2 horizontal, 2 perpendicular
  measures "d87" distance of L2.end L3.end
  measures "d88" distance of L1.end L2.end
  measures "d91" distance between parallel lines of L5 L4
  measures "d92" distance between parallel lines of L0 L1
  measures "d93" distance between parallel lines of L2 L7
  measures "d94" distance of L6.start L6.end
  measures "d95" distance of L6.end L7.end
  measures "d96" distance between parallel lines of L0 L8
extrude "Vysunutí7" cut sketch "Náčrt10" against normal through all
sketch "Náčrt11" plane through (0, 3, 0) normal (0, 1, 0) x (1, 0, 0)
  circle A0 centre (43, 59) radius 1.5
  circle A1 centre (43, 41) radius 1.5
  line L0 (137, 3) -> (13, 3) projected
  line L1 (13, 97) -> (137, 97) projected
  line L2 (3, 13) -> (3, 87) projected
  point P0 (0, 0)
  dimension "d99" = 3
  dimension "d100" = 3
  dimension "d101" = 38
  dimension "d102" = 38
  dimension "d103" = 40
  dimension "d104" = 40
  constraints: 2 centre point
  measures "d99" diameter of A0
  measures "d100" diameter of A1
  measures "d101" distance from line of L0 A1.centre
  measures "d102" distance from line of L1 A0.centre
  measures "d103" distance from line of L2 A0.centre
  measures "d104" distance from line of L2 A1.centre
extrude "Vysunutí8" add sketch "Náčrt11" along normal blind 11
sketch "Náčrt12" plane through (3, 50, -13) normal (1, 0, 0) x (0, 0, -1)
  circle A0 centre (37, -42) radius 3.5
  line L0 (0, -47) -> (74, -47) projected
  line L1 (74, 0) -> (74, -47) projected
  point P0 (-13, -50)
  point P1 (74, -50)
  dimension "d107" = 7
  dimension "d108" = 5
  constraints: 1 centre point
  measures "d107" diameter of A0
  measures "d108" distance from line of A0.centre L0
extrude "Vysunutí9" cut sketch "Náčrt12" against normal through all
sketch "Náčrt13" plane through (0, 3, 0) normal (0, 1, 0) x (1, 0, 0)
  line L0 (147, 87) -> (147, 13) projected
  circle A0 centre (118, 81) radius 1
  circle A1 centre (137, 81) radius 1
  circle A2 centre (118, 42) radius 1
  circle A3 centre (137, 42) radius 1
  point P0 (0, 0)
  dimension "d115" = 2
  dimension "d116" = 2
  constraints: 4 centre point
  measures "d115" diameter of A0
  measures "d116" diameter of A1
extrude "Vysunutí10" add sketch "Náčrt13" along normal blind 10
